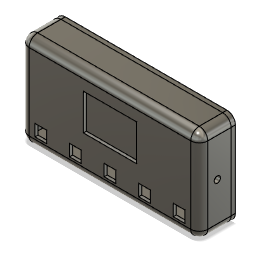
LED Display v1 (Autodesk Fusion 360 design; units mm, degrees)
Autodesk Fusion 360 part; units mm, degrees
box "BoxPrimitive1" add length 44 width 84 height 17 placed x (0, 1, 0) y (-1, 0, 0) z (0, 0, 1) at (84, 0, 0) makes body 1
shell "Shell1" thickness 2 removed faces 0 bodies 1
ref_plane "WorkPlane1" through (42, 22, 2) normal (0, 0, -1) x (0, -1, 0)
split "Split1" by plane through (42, 22, 2) normal (0, 0, -1) bodies 1 makes body 2 at (28, 14.6667, 0)
sketch "Sketch2" plane through (0, 0, 17) normal (0, 0, 1) x (-1, 0, 0)
  line L0 (-2, 42) -> (-82, 42)
  line L1 (-82, 42) -> (-82, 2)
  line L2 (-82, 2) -> (-2, 2)
  line L3 (-2, 2) -> (-2, 42)
  line L4 (-42, 42) -> (-42, 35)
  line L5 (-42, 35) -> (-42, 18)
  line L6 (-42, 18) -> (-29.5, 18)
  line L7 (-29.5, 18) -> (-54.5, 18)
  line L8 (-54.5, 18) -> (-54.5, 35)
  line L9 (-54.5, 35) -> (-29.5, 35)
  line L10 (-29.5, 35) -> (-29.5, 18)
  line L11 (-42, 18) -> (-42, 10.5)
  line L12 (-42, 10.5) -> (-42, 7.75)
  line L13 (-39.25, 10.5) -> (-44.75, 10.5)
  line L14 (-44.75, 10.5) -> (-44.75, 5)
  line L15 (-44.75, 5) -> (-39.25, 5)
  line L16 (-39.25, 5) -> (-39.25, 10.5)
  line L17 (-39.25, 10.5) -> (-44.75, 5) construction
  line L18 (-44.75, 10.5) -> (-39.25, 5) construction
  line L19 (-42, 7.75) -> (-6.75, 7.75)
  line L20 (-71.75, 10.5) -> (-77.25, 10.5)
  line L21 (-77.25, 10.5) -> (-77.25, 5)
  line L22 (-77.25, 5) -> (-71.75, 5)
  line L23 (-71.75, 5) -> (-71.75, 10.5)
  line L24 (-55.5, 10.5) -> (-61, 10.5)
  line L25 (-61, 10.5) -> (-61, 5)
  line L26 (-61, 5) -> (-55.5, 5)
  line L27 (-55.5, 5) -> (-55.5, 10.5)
  line L28 (-23, 10.5) -> (-28.5, 10.5)
  line L29 (-28.5, 10.5) -> (-28.5, 5)
  line L30 (-28.5, 5) -> (-23, 5)
  line L31 (-23, 5) -> (-23, 10.5)
  line L32 (-6.75, 10.5) -> (-12.25, 10.5)
  line L33 (-12.25, 10.5) -> (-12.25, 5)
  line L34 (-12.25, 5) -> (-6.75, 5)
  line L35 (-6.75, 5) -> (-6.75, 10.5)
  line L36 (-84, -44) -> (0, -44)
  line L37 (0, -44) -> (0, 0)
  line L38 (0, 0) -> (-84, 0)
  line L39 (-84, 0) -> (-84, -44)
  line L40 (-61, -5) -> (-55.5, -5)
  line L41 (-42, -42) -> (-42, -35)
  line L42 (-54.5, -18) -> (-54.5, -35)
  line L43 (-54.5, -35) -> (-29.5, -35)
  line L44 (-42, -18) -> (-42, -10.5)
  line L45 (-44.75, -10.5) -> (-44.75, -5)
  line L46 (-2, -42) -> (-82, -42)
  line L47 (-44.75, -10.5) -> (-39.25, -5) construction
  line L48 (-82, -2) -> (-2, -2)
  line L49 (-39.25, -10.5) -> (-44.75, -5) construction
  line L50 (-77.25, -10.5) -> (-77.25, -5)
  line L51 (-12.25, -10.5) -> (-12.25, -5)
  line L52 (-29.5, -35) -> (-29.5, -18)
  line L53 (-71.75, -10.5) -> (-77.25, -10.5)
  line L54 (-23, -5) -> (-23, -10.5)
  line L55 (-71.75, -5) -> (-71.75, -10.5)
  line L56 (-77.25, -5) -> (-71.75, -5)
  line L57 (-42, -35) -> (-42, -18)
  line L58 (-23, -10.5) -> (-28.5, -10.5)
  line L59 (-28.5, -10.5) -> (-28.5, -5)
  line L60 (-55.5, -5) -> (-55.5, -10.5)
  line L61 (-61, -10.5) -> (-61, -5)
  line L62 (-6.75, -5) -> (-6.75, -10.5)
  line L63 (-82, -42) -> (-82, -2)
  line L64 (-44.75, -5) -> (-39.25, -5)
  line L65 (-6.75, -10.5) -> (-12.25, -10.5)
  line L66 (-29.5, -18) -> (-54.5, -18)
  line L67 (-2, -2) -> (-2, -42)
  line L68 (-55.5, -10.5) -> (-61, -10.5)
  line L69 (-42, -10.5) -> (-42, -7.75)
  line L70 (-28.5, -5) -> (-23, -5)
  line L71 (-42, -7.75) -> (-6.75, -7.75)
  line L72 (-42, -18) -> (-29.5, -18)
  line L73 (-39.25, -5) -> (-39.25, -10.5)
  line L74 (-12.25, -5) -> (-6.75, -5)
  line L75 (-39.25, -10.5) -> (-44.75, -10.5)
  line L76 (-2.25, -41.75) -> (-81.75, -41.75)
  line L77 (-81.75, -41.75) -> (-81.75, -2.25)
  line L78 (-81.75, -2.25) -> (-2.25, -2.25)
  line L79 (-2.25, -2.25) -> (-2.25, -41.75)
  point P0 (-42, 7.75)
  point P1 (-42, -7.75)
  dimension "d8" = 12.5
  dimension "d9" = 25
  dimension "d10" = 17
  dimension "d11" = 7.5
  dimension "d12" = 2.75
  dimension "d13" = 5.5
  dimension "d14" = 5.5
  dimension "d15" = 35.25
  dimension "d18" = 32.5
  dimension "d19" = 0
  dimension "d22" = 0.25
  constraint midpoint L0 L4.start
  constraint perpendicular L0 L4
  constraint perpendicular L0 L5
  constraint perpendicular L5 L6
  constraint horizontal L7
  constraint vertical L8
  constraint horizontal L9
  constraint vertical L10
  constraint perpendicular L7 L11
  constraint parallel L11 L12
  constraint horizontal L13
  constraint perpendicular L13 L14
  constraint parallel L13 L15
  constraint parallel L14 L16
  constraint coincident L17 P0
  constraint coincident L18 P0
  constraint coincident P0 L12.end
  constraint perpendicular L12 L19
  constraint symmetric L0.start L38 L46.start
  constraint symmetric L0.end L38 L46.end
  constraint symmetric L1.end L38 L48.start
  constraint symmetric L2.end L38 L48.end
  constraint symmetric L4.start L38 L41.start
  constraint symmetric L4.end L38 L41.end
  constraint symmetric L5.end L38 L44.start
  constraint symmetric L6.end L38 L52.end
  constraint symmetric L7.end L38 L42.start
  constraint symmetric L8.end L38 L42.end
  constraint symmetric L9.end L38 L43.end
  constraint symmetric L11.end L38 L44.end
  constraint symmetric P0 L38 P1
  constraint symmetric L13.start L38 L49.start
  constraint symmetric L13.end L38 L45.start
  constraint symmetric L14.end L38 L45.end
  constraint symmetric L15.end L38 L47.end
  constraint symmetric L19.end L38 L71.end
  constraint symmetric L20.start L38 L53.start
  constraint symmetric L20.end L38 L50.start
  constraint symmetric L21.end L38 L50.end
  constraint symmetric L22.end L38 L55.start
  constraint symmetric L24.start L38 L60.end
  constraint symmetric L24.end L38 L61.start
  constraint symmetric L25.end L38 L40.start
  constraint symmetric L26.end L38 L40.end
  constraint symmetric L28.start L38 L54.end
  constraint symmetric L28.end L38 L58.end
  constraint symmetric L29.end L38 L59.end
  constraint symmetric L30.end L38 L54.start
  constraint symmetric L32.start L38 L62.end
  constraint symmetric L32.end L38 L51.start
  constraint symmetric L33.end L38 L51.end
  constraint symmetric L34.end L38 L62.start
  measures "d8" distance of L5.end L6.end
  measures "d9" distance of L6.end L7.end
  measures "d10" distance of L6.end L9.end
  measures "d11" distance of L5.end L11.end
  measures "d12" distance of L11.end P0
  measures "d13" distance of L14.end L15.end
  measures "d14" distance of L13.end L14.end
  measures "d15" distance of P0 L19.end
extrude "Extrude2" add sketch "Sketch2" along normal blind -16 and the other way blind 13 contours L40 L60 L61 L68 | L42 L43 L57 L66 | L43 L52 L57 L66 L72 | L45 L64 L69 L71 L73 L75 | L69 L71 L73 L75 | L50 L53 L55 L56 | L51 L62 L65 L71 | L51 L62 L71 L74 | L54 L59 L70 L71 | L54 L58 L59 L71 | L76 L77 L78 L79 bodies 2
extrude "Extrude1" cut sketch "Sketch2" against normal blind 2 draft 15 contours L40 L60 L61 L68 | L42 L43 L57 L66 | L43 L52 L57 L66 L72 | L45 L64 L69 L71 L73 L75 | L69 L71 L73 L75 | L50 L53 L55 L56 | L51 L62 L65 L71 | L51 L62 L71 L74 | L54 L59 L70 L71 | L54 L58 L59 L71 bodies 1
fillet "Fillet1" radius 4 12 edges at (0, 44, 9.5) (84, 44, 9.5) (0, 0, 9.5) (84, 0, 9.5) (42, 0, 17) (42, 44, 17) (84, 22, 17) (0, 22, 17) (0, 44, 1) (84, 44, 1) (0, 0, 1) (84, 0, 1) on bodies 1 2
hole "Hole1" at (82, 22, 8.5) direction (1, 0, 0) diameter 3 depth 14 tip angle 118 bodies 1
equation "d8 = ( 25 / 2 ) * 1 mm"
equation "d12 = ( 5.5 / 2 ) * 1 mm"
equation "d15 = ( 70.5 / 2 ) * 1 mm"
